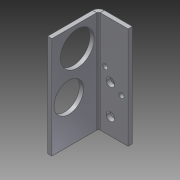
# Autodesk Inventor part: Shooter Magnetic Sensor Mount Bracket
Saved by Autodesk Inventor 2014 SP1 (Build 180222100, 222)
## iProperties
Created: 2013-12-15
Part Number: Shooter Magnetic Sensor Mount Bracket
Material: Aluminum 6061
Document SubType Name: Sheet Metal
Designer: Moses
Density: 2.71 g/cm^3
Sheet Metal Rule: Default
Appearance: Aluminum - Flat
Mass: 30.3086 g
Surface Area: 85.8189 cm^2
Volume: 11.184 cm^3
Author: Moses
Autodesk Inventor part; units mm, degrees
ref_plane "YZ Plane" through (0, 0, 0) normal (1, 0, 0) x (0, 1, 0)
ref_plane "XZ Plane" through (0, 0, 0) normal (0, 1, 0) x (-1, 0, 0)
ref_plane "XY Plane" through (0, 0, 0) normal (0, 0, 1) x (1, 0, 0)
sketch "Sketch1" plane through (0, 0, 0) normal (0, 0, 1) x (1, 0, 0)
  line L0 (0, 0) -> (25.4, 0)
  line L1 (25.4, 0) -> (25.4, 76.2)
  line L2 (25.4, 76.2) -> (0, 76.2)
  line L3 (0, 76.2) -> (0, 0)
  dimension "d0" = 25.4
  dimension "d1" = 76.2
  measures "d0" distance of L2.end L1.end
  measures "d1" distance of L1.end L0.end
extrude "Plate1" add sketch "Sketch1" along normal blind 3.175
sketch "Sketch2" plane through (3.175, 0, 0) normal (-1, 0, 0) x (0, -1, 0)
  line L0 (-76.2, 0) -> (0, 0)
  line L1 (0, 0) -> (0, 38.1)
  line L2 (0, 38.1) -> (-76.2, 38.1)
  line L3 (-76.2, 38.1) -> (-76.2, 0)
  constraints: 6 end point, 1 horizontal, 1 perpendicular, 1 vertical
edge flange "Flange1" height 38.1 angle 90 thickness 3.175 bend radius 1.27 thickness toward (-1, 0, 0) relief tear relief width 3.175 relief depth 1.5875 edges at (0, 38.1, 3.175) wall of the first edge with corners at (3.175, 76.2, 0) (3.175, 0, 0) (3.175, 0, 38.1) (3.175, 76.2, 38.1)
bend "Bend1"
corner "Corner1"
sketch "Sketch3" plane through (0, 0, 38.1) normal (-1, 0, 0) x (0, 0, 1)
  line L0 (0, 0) -> (-33.655, 0) projected
  line L1 (0, 76.2) -> (0, 0) projected
  line L2 (-33.655, 76.2) -> (0, 76.2) projected
  circle A0 centre (-19.05, 60.325) radius 12.7
  circle A1 centre (-12.7, 31.75) radius 11.1125
  point P0 (-38.1, 0)
  dimension "d13" = 25.4
  dimension "d14" = 22.225
  dimension "d15" = 15.875
  dimension "d16" = 19.05
  dimension "d17" = 12.7
  dimension "d18" = 31.75
  constraints: 2 centre point
  measures "d13" diameter of A0
  measures "d14" diameter of A1
  measures "d15" distance from line of A0.centre L2
  measures "d16" distance from line of A0.centre L1
  measures "d17" distance from line of A1.centre L1
  measures "d18" distance from line of L0 A1.centre
extrude "Cut1" cut sketch "Sketch3" against normal blind 3.175
sketch "Sketch4" plane through (0, 0, 3.175) normal (0, 0, 1) x (1, 0, 0)
  line L0 (4.445, 76.2) -> (4.445, 0) projected
  line L1 (25.4, 76.2) -> (25.4, 0) projected
  circle A0 centre (-69.6884, -88.0779) radius 3.3782 construction
  circle A1 centre (-79.6289, 46.8501) radius 3.3782 construction
  circle A2 centre (-113.1559, 49.7834) radius 3.3782 construction
  circle A3 centre (-43.9071, -66.4449) radius 3.3782 construction
  line L2 (-118.5182, 63.001) -> (-315.8997, 80.2697) construction
  arc A4 (-315.8997, 80.2697) -> (-318.1134, 54.9663) centre (74.9912, 33.3226) ccw construction
  line L3 (-318.1134, 54.9663) -> (38.1, 23.8017) construction
  arc A5 (38.1, 23.8017) -> (42.1314, 14.0393) centre (74.9912, 33.3226) ccw construction
  line L4 (42.1314, 14.0393) -> (-230.643, -214.8455) construction
  arc A6 (-230.643, -214.8455) -> (-226.6005, -219.7429) centre (74.9912, 33.3226) ccw construction
  line L5 (-226.6005, -219.7429) -> (-222.5188, -224.6072) construction
  line L6 (-222.5188, -224.6072) -> (50.2948, 4.3106) construction
  arc A7 (50.2948, 4.3106) -> (55.7079, 66.1824) centre (74.9912, 33.3226) ccw construction
  line L7 (55.7079, 66.1824) -> (15.7878, 113.7573) construction
  arc A8 (-3.434, 116.9073) -> (15.7878, 113.7573) centre (29.7432, 259.139) ccw construction
  line L8 (-3.434, 116.9073) -> (-110.1078, 141.7901) construction
  line L9 (-110.1078, 141.7901) -> (-116.0889, 251.1642) construction
  arc A9 (-115.8532, 270.641) -> (-116.0889, 251.1642) centre (29.7432, 259.139) ccw construction
  line L10 (-115.8532, 270.641) -> (-173.2099, 338.996) construction
  line L11 (-173.2099, 338.996) -> (-178.0743, 334.9143) construction
  arc A10 (-178.0743, 334.9143) -> (-182.9057, 330.7934) centre (74.9912, 33.3226) ccw construction
  line L12 (-182.9057, 330.7934) -> (-129.6946, 267.3788) construction
  line L13 (-129.6946, 267.3788) -> (-118.5182, 63.001) construction
  circle A11 centre (-173.9926, 330.0499) radius 3.3782 construction
  circle A12 centre (-141.339, 291.1349) radius 3.3782 construction
  line L14 (-105.7381, 61.8829) -> (-109.3854, 128.5807) construction
  line L15 (-109.3854, 128.5807) -> (10.1717, 100.6927) construction
  line L16 (10.1717, 100.6927) -> (45.9792, 58.019) construction
  arc A13 (45.9792, 58.019) -> (40.3138, 49.105) centre (74.9912, 33.3226) ccw construction
  line L17 (40.3138, 49.105) -> (-105.7381, 61.8829) construction
  circle A14 centre (74.9912, 33.3226) radius 9.5 construction
  circle A15 centre (-310.4012, 72.216) radius 3.3782 construction
  circle A16 centre (-311.3, 61.9429) radius 3.3782 construction
  circle A17 centre (-259.7945, 67.7885) radius 3.3782 construction
  circle A18 centre (-260.6933, 57.5153) radius 3.3782 construction
  circle A19 centre (-221.7361, -215.6611) radius 3.3782 construction
  circle A20 centre (-182.821, -183.0075) radius 3.3782 construction
  circle A21 centre (-32.0252, -56.4748) radius 3.3782 construction
  circle A22 centre (-139.0416, -146.2722) radius 3.3782 construction
  circle A23 centre (-63.4799, 51.8115) radius 3.3782 construction
  circle A24 centre (-64.5868, 39.1599) radius 3.3782 construction
  circle A25 centre (-202.7203, 63.9935) radius 3.3782 construction
  circle A26 centre (-203.8271, 51.3418) radius 3.3782 construction
  circle A27 centre (20.32, 30.4566) radius 1.905
  circle A28 centre (8.255, 43.1566) radius 1.905
  line L18 (25.4, 0) -> (4.445, 0) projected
  line L19 (4.445, 76.2) -> (25.4, 76.2) projected
  line L20 (12.065, 76.2) -> (12.065, 0) construction
  circle A29 centre (12.065, 12.7) radius 3.175
  circle A30 centre (12.065, 34.925) radius 3.175
  point P0 (0, 0)
  dimension "d21" = 3.81
  dimension "d22" = 5.08
  dimension "d23" = 5.08
  dimension "d24" = 12.7
  dimension "d25" = 3.81
  dimension "d28" = 7.62
  dimension "d29" = 6.35
  dimension "d30" = 12.7
  dimension "d31" = 22.225
  constraints: 4 centre point, 4 point on line, 2 end point, 2 equal radius, 1 vertical
  measures "d21" diameter of A27
  measures "d22" distance from line of L3 A27.centre
  measures "d23" distance from line of L1 A27.centre
  measures "d24" vertical distance of A27.centre A28.centre
  measures "d25" distance from line of L0 A28.centre
  measures "d28" distance between parallel lines of L20 L0
  measures "d29" diameter of A29
  measures "d30" distance from line of L18 A29.centre
  measures "d31" distance of A29.centre A30.centre
extrude "Cut2" cut sketch "Sketch4" against normal blind 3.175 contours A27 | A28 | A29 | A30
equation "\"d19\" = Thickness"
equation "\"d26\" = Thickness"
equation "\"d3\" = BendReliefWidth"
equation "\"d4\" = BendReliefDepth"
equation "\"d5\" = MinimumRemnant"
equation "\"d6\" = BendRadius"
equation "\"d10\" = CornerReliefSize"
equation "\"d11\" = GapSize"
equation "\"d12\" = JacobiRadiusSize"
equation "\"BendRadius\" = Thickness"
equation "\"BendReliefWidth\" = Thickness"
equation "\"BendReliefDepth\" = 0.5 * Thickness"
equation "\"CornerReliefSize\" = 4 * Thickness"
equation "\"MinimumRemnant\" = 2 * Thickness"
equation "\"TransitionRadius\" = BendRadius"
equation "\"JacobiRadiusSize\" = BendRadius"
equation "\"GapSize\" = Thickness"
equation "\"d2\" = BendRadius"
equation "\"Thickness\" = 3.175"
body "Solid1"
